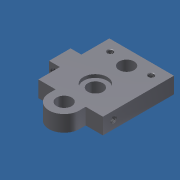
# Autodesk Inventor part: PLACA COM FUROS COORDENADOS(13)
Saved by Autodesk Inventor 2012 SP1 (Build 160190100, 190)
## iProperties
Created: 2012-07-23
Part Number: PLACA COM FUROS COORDENADOS(13)
Material: Carbon Steel
Document SubType Name: Modeling
Designer: bruno.silveira
Mass: 609.138 g
Surface Area: 147 cm^2
Volume: 77.4 cm^3
Density: 7.87 g/cm^3
Author: bruno.silveira
Autodesk Inventor part; units mm, degrees
ref_plane "YZ Plane" through (0, 0, 0) normal (1, 0, 0) x (0, 1, 0)
ref_plane "XZ Plane" through (0, 0, 0) normal (0, 1, 0) x (-1, 0, 0)
ref_plane "XY Plane" through (0, 0, 0) normal (0, 0, 1) x (1, 0, 0)
sketch "Sketch1" plane through (0, 0, 0) normal (0, 0, 1) x (1, 0, 0)
  line L0 (0, 0) -> (80, 0)
  line L1 (80, 0) -> (80, 86)
  line L2 (80, 86) -> (0, 86)
  line L3 (0, 86) -> (0, 0)
  dimension "d0" = 80
  dimension "d1" = 86
  constraints: 8 end point, 2 parallel, 1 horizontal, 1 perpendicular
  measures "d0" distance of L1.end L2.end
  measures "d1" distance of L0.end L1.end
extrude "Extrusion1" add sketch "Sketch1" along normal blind 15
sketch "Sketch2" plane through (0, 0, 15) normal (0, 0, 1) x (1, 0, 0)
  line L0 (0, 0) -> (0, 86) projected
  line L1 (80, 0) -> (0, 0) projected
  line L2 (80, 86) -> (80, 0) projected
  line L3 (0, 86) -> (80, 86) projected
  line L4 (0, 86) -> (10, 86)
  line L5 (10, 86) -> (10, 60)
  line L6 (10, 60) -> (0, 60)
  line L7 (0, 60) -> (0, 86)
  line L8 (70, 86) -> (80, 86)
  line L9 (80, 86) -> (80, 40)
  line L10 (80, 40) -> (70, 40)
  line L11 (70, 40) -> (70, 86)
  line L12 (54, 0) -> (80, 0)
  line L13 (80, 0) -> (80, 20)
  line L14 (80, 20) -> (54, 20)
  line L15 (54, 20) -> (54, 0)
  line L16 (0, 20) -> (26, 20)
  line L17 (26, 20) -> (26, 0)
  line L18 (26, 0) -> (0, 0)
  line L19 (0, 0) -> (0, 20)
  dimension "d4" = 20
  dimension "d5" = 20
  dimension "d6" = 20
  dimension "d7" = 10
  dimension "d8" = 10
  dimension "d9" = 40
  dimension "d10" = 28
  dimension "d11" = 26
  constraints: 32 end point, 8 parallel, 6 point on line, 4 horizontal, 4 perpendicular
  measures "d4" distance of L16.end L17.end
  measures "d5" distance of L14.end L12.start
  measures "d6" distance between parallel lines of L14 L10
  measures "d7" distance of L9.end L10.end
  measures "d8" distance of L5.end L6.end
  measures "d9" distance between parallel lines of L16 L6
  measures "d10" distance between parallel lines of L15 L17
  measures "d11" distance between parallel lines of L0 L17
extrude "Extrusion2" cut sketch "Sketch2" against normal blind 15 contours L0 L16 L17 L1 | L0 L3 L5 L6 | L15 L14 L2 L1 | L3 L2 L10 L11
sketch "Sketch3" plane through (0, 0, 15) normal (0, 0, 1) x (1, 0, 0)
  line L0 (10, 86) -> (10, 60) projected
  line L1 (10, 60) -> (0, 60) projected
  line L2 (0, 20) -> (0, 60) projected
  line L3 (0, 20) -> (26, 20) projected
  line L4 (26, 20) -> (26, 0) projected
  line L5 (54, 0) -> (26, 0) projected
  line L6 (54, 0) -> (54, 20) projected
  line L7 (54, 20) -> (80, 20) projected
  line L8 (80, 40) -> (80, 20) projected
  line L9 (80, 40) -> (70, 40) projected
  line L10 (70, 40) -> (70, 86) projected
  line L11 (10, 86) -> (70, 86) projected
  line L12 (0, 20) -> (10, 20)
  line L13 (10, 20) -> (10, 40)
  line L14 (10, 40) -> (0, 40)
  line L15 (0, 40) -> (0, 20)
  point P0 (0, 0)
  dimension "d14" = 10
  dimension "d15" = 20
  constraints: 8 end point, 2 parallel, 1 horizontal, 1 perpendicular
  measures "d14" distance of L13.end L14.end
  measures "d15" distance of L12.end L13.end
extrude "Extrusion3" cut sketch "Sketch3" against normal blind 15 contours L14 L13 L3 L2
sketch "Sketch4" plane through (0, 0, 15) normal (0, 0, 1) x (1, 0, 0)
  line L0 (26, 20) -> (26, 0) projected
  line L1 (54, 0) -> (26, 0) projected
  line L2 (10, 86) -> (70, 86) projected
  line L3 (0, 40) -> (0, 60) projected
  point P0 (0, 0)
  point P1 (40, 72)
  point P2 (40, 14)
  dimension "d18" = 14
  dimension "d19" = 40
  dimension "d20" = 14
  dimension "d21" = 14
  measures "d18" distance from line of L2 point (40, 72)
  measures "d19" distance from line of L3 point (40, 72)
  measures "d20" distance from line of L1 point (40, 14)
  measures "d21" distance from line of L0 point (40, 14)
hole "Hole1" at (40, 72, 15) at (40, 14, 15) direction (0, 0, -1) diameter 14 depth 15 tip angle 118
sketch "Sketch5" plane through (0, 0, 15) normal (0, 0, 1) x (1, 0, 0)
  circle A0 centre (40, 72) radius 7 projected
  line L0 (0, 40) -> (0, 60) projected
  point P0 (0, 0)
  point P1 (40, 43)
  dimension "d29" = 29
  dimension "d30" = 40
  measures "d29" distance of A0.centre point (40, 43)
  measures "d30" distance from line of L0 point (40, 43)
hole "Hole2" at (40, 43, 15) direction (0, 0, -1) diameter 14 depth 18 tip angle 118 counterbore diameter 22 counterbore depth 3
fillet "Fillet1" radius 14 2 edges at (26, 0, 7.5) (54, 0, 7.5)
sketch "Sketch6" plane through (0, 0, 15) normal (0, 0, 1) x (1, 0, 0)
  line L0 (70, 40) -> (80, 40)
  line L1 (80, 40) -> (80, 20)
  line L2 (80, 20) -> (70, 20)
  line L3 (70, 20) -> (70, 40)
  point P0 (0, 0)
  constraints: 8 end point, 2 parallel, 1 horizontal, 1 perpendicular
extrude "Extrusion4" cut sketch "Sketch6" against normal blind 15
sketch "Sketch7" plane through (0, 60, 15) normal (0, 1, 0) x (1, 0, 0)
  line L0 (0, 15) -> (10, 15) projected
  line L1 (10, 0) -> (10, 15) projected
  point P0 (5, 7.5)
  dimension "d41" = 7.5
  dimension "d42" = 5
  measures "d41" distance from line of L0 point (5, 7.5)
  measures "d42" distance from line of L1 point (5, 7.5)
hole "Hole3" at (5, 60, 7.5) direction (0, -1, 0) diameter 6.647 depth 20 tip angle 118 thread size "M8x1.25" class "6H" standard "ANSI Metric M Profile"
chamfer "Chamfer1" distance 0.5 angle 45 2 edges at (5, 60, 4.1765) (5, 40, 4.1765)
sketch "Sketch8" plane through (0, 0, 15) normal (0, 0, 1) x (1, 0, 0)
  circle A0 centre (40, 72) radius 7 projected
  line L0 (10, 86) -> (70, 86) projected
  point P0 (0, 0)
  point P1 (21, 76)
  point P2 (59, 76)
  dimension "d53" = 38
  dimension "d54" = 19
  dimension "d55" = 10
  measures "d53" distance of point (21, 76) point (59, 76)
  measures "d54" horizontal distance of A0.centre point (21, 76)
  measures "d55" distance from line of L0 point (21, 76)
hole "Hole4" at (21, 76, 15) at (59, 76, 15) direction (0, 0, -1) diameter 4.917 depth 12 tip angle 118 thread size "M6x1" class "6H" standard "ANSI Metric M Profile"
chamfer "Chamfer2" distance 0.5 angle 45 2 edges at (21, 78.4585, 15) (59, 78.4585, 15)
sketch "Sketch9" plane through (70, 20, 15) normal (1, 0, 0) x (0, 0, -1)
  line L0 (15, 66) -> (15, 0) projected
  line L1 (0, 66) -> (15, 66) projected
  point P0 (15, -20)
  point P1 (7.5, 10)
  dimension "d66" = 7.5
  dimension "d67" = 56
  measures "d66" distance from line of L0 point (7.5, 10)
  measures "d67" distance from line of L1 point (7.5, 10)
hole "Hole5" at (70, 30, 7.5) direction (-1, 0, 0) diameter 4.917 depth 15 tip angle 118 thread size "M6x1" class "6H" standard "ANSI Metric M Profile"
chamfer "Chamfer3" distance 0.5 angle 45 1 edges at (70, 30, 9.9585)
sketch "Sketch10" plane through (10, 20, 15) normal (-1, 0, 0) x (0, 0, 1)
  line L0 (-15, 0) -> (-15, 20) projected
  line L1 (0, 0) -> (-15, 0) projected
  point P0 (-15, -20)
  point P1 (-7.5, 10)
  dimension "d78" = 10
  dimension "d79" = 7.5
  measures "d78" distance from line of L1 point (-7.5, 10)
  measures "d79" distance from line of L0 point (-7.5, 10)
hole "Hole6" at (10, 30, 7.5) direction (1, 0, 0) diameter 4.917 depth 15 tip angle 118 thread size "M6x1" class "6H" standard "ANSI Metric M Profile"
chamfer "Chamfer4" distance 0.5 angle 45 1 edges at (10, 30, 5.0415)
body "Solid1"
